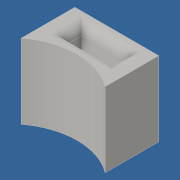
# Autodesk Inventor part: vibramount
Saved by Autodesk Inventor 2016 (Build 200138000, 138)
## iProperties
Created: 2017-05-29
Part Number: vibramount
Material: Generisch
Document SubType Name: Modeling
Designer: 4ndreas
Density: 1 g/cm^3
Appearance: Vorgabe
Author: 4ndreas
Autodesk Inventor part; units mm, degrees
ref_plane "YZ Plane" through (0, 0, 0) normal (1, 0, 0) x (0, 1, 0)
ref_plane "XZ Plane" through (0, 0, 0) normal (0, 1, 0) x (-1, 0, 0)
ref_plane "XY Plane" through (0, 0, 0) normal (0, 0, 1) x (1, 0, 0)
sketch "Skizze1" plane through (0, 0, 0) normal (0, 0, 1) x (1, 0, 0)
  line L0 (-5, -1.75) -> (5, -1.75)
  line L1 (5, -1.75) -> (5, 1.75)
  line L2 (5, 1.75) -> (-5, 1.75)
  line L3 (-5, 1.75) -> (-5, -1.75)
  line L4 (-5, -1.75) -> (5, 1.75) construction
  line L5 (5, -1.75) -> (-5, 1.75) construction
  line L6 (-9, -4.25) -> (9, -4.25)
  line L7 (9, -4.25) -> (9, 4.25)
  line L8 (9, 4.25) -> (-9, 4.25)
  line L9 (-9, 4.25) -> (-9, -4.25)
  line L10 (-9, -4.25) -> (9, 4.25) construction
  line L11 (9, -4.25) -> (-9, 4.25) construction
  line L12 (-9, -4.25) -> (-9, -7.25)
  line L13 (9, -4.25) -> (9, -7.25)
  arc A0 (9, -7.25) -> (-9, -7.25) centre (0, -19.25) ccw
  point P0 (0, 0)
  dimension "d0" = 10
  dimension "d1" = 3.5
  dimension "d2" = 18
  dimension "d3" = 2.5
  dimension "d4" = 3
  constraints: 28 end point, 5 parallel, 4 midpoint, 2 horizontal, 2 perpendicular, 2 point on circle, 2 vertical, 1 centre point, 1 tangent
  measures "d0" distance between parallel lines of L1 L3
  measures "d1" distance between parallel lines of L0 L2
  measures "d2" distance between parallel lines of L7 L9
  measures "d3" distance between parallel lines of L2 L8
  measures "d4" distance of L6.start L12.end
extrude "Extrusion1" add sketch "Skizze1" along normal blind 13
sketch "Skizze2" plane through (0, 0, 0) normal (0, 0, -1) x (-1, 0, 0)
  line L0 (5, 1.75) -> (5, -1.75) projected
  line L1 (5, -1.75) -> (-5, -1.75) projected
  line L2 (-5, -1.75) -> (-5, 1.75) projected
  line L3 (-5, 1.75) -> (5, 1.75) projected
  line L4 (9, 4.25) -> (9, -7.25) projected
  line L5 (-9, 4.25) -> (9, 4.25) projected
  line L6 (-9, -7.25) -> (-9, 4.25) projected
  arc A0 (9, -7.25) -> (-9, -7.25) centre (0, -19.25) ccw projected
  point P0 (0, 0)
extrude "Extrusion2" add sketch "Skizze2" along normal blind 3 contours L0 L1 L2 L3 | L4 A0 L6 L5
fillet "Rundung1" radius 2 4 edges at (-5, 0, 13) (5, 0, 13) (0, 1.75, 13) (0, -1.75, 13)
